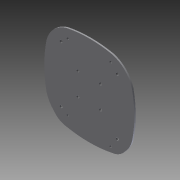
# Autodesk Inventor part: Base
Saved by Autodesk Inventor 2011 SP1 (Build 150282100, 282)
## iProperties
Created: 2011-07-18
Part Number: Base
Document SubType Name: Modeling
Designer: Nathan
Density: 1 g/cm^3
Author: Nathan
Autodesk Inventor part; units mm, degrees
ref_plane "YZ Plane" through (0, 0, 0) normal (1, 0, 0) x (0, 1, 0)
ref_plane "XZ Plane" through (0, 0, 0) normal (0, 1, 0) x (-1, 0, 0)
ref_plane "XY Plane" through (0, 0, 0) normal (0, 0, 1) x (1, 0, 0)
sketch "Sketch1" plane through (0, 0, 0) normal (0, 0, 1) x (1, 0, 0)
  line L0 (0, 3.1673) -> (0, -2.4908)
  spline S0 degree 2 poles (-48.26, -25.4) (-53.34, 0) (-48.26, 25.4) knots 0 0 0 1 1 1
  line L1 (-20.5368, 0) -> (25.7294, 0)
  line L2 (0, 0) -> (-9.8402, -9.8402)
  line L3 (0, 0) -> (13.9161, 0) construction
  line L4 (0, 0) -> (-23.2805, 23.2805)
  arc A0 (-39.9068, 39.9068) -> (-48.26, 25.4) centre (-17.1376, 17.1376) ccw
  arc A1 (-48.26, -25.4) -> (-39.9068, -39.9068) centre (-17.1376, -17.1376) ccw
  spline S1 degree 2 poles (48.26, -25.4) (53.34, 0) (48.26, 25.4) knots 0 0 0 1 1 1
  arc A2 (48.26, 25.4) -> (39.9068, 39.9068) centre (17.1376, 17.1376) ccw
  arc A3 (39.9068, -39.9068) -> (48.26, -25.4) centre (17.1376, -17.1376) ccw
  spline S2 degree 2 poles (25.476, -48.26) (-0.0768, -53.34) (-25.476, -48.26) knots 0 0 0 1 1 1
  arc A4 (-39.9068, -39.9068) -> (-25.476, -48.26) centre (-23.264, -27.7968) ccw
  arc A5 (25.476, -48.26) -> (39.9068, -39.9068) centre (23.264, -27.7968) ccw
  spline S3 degree 2 poles (-25.4, 48.26) (0, 53.34) (25.4, 48.26) knots 0 0 0 1 1 1
  arc A6 (39.9068, 39.9068) -> (25.4, 48.26) centre (17.1376, 17.1376) ccw
  arc A7 (-25.4, 48.26) -> (-39.9068, 39.9068) centre (-17.1376, 17.1376) ccw
  point P0 (-50.8, 0)
  point P1 (50.8, 0)
  point P2 (-0.076, -50.8)
  point P3 (0, 50.8)
  point P4 (-12.7, 12.7)
  point P5 (-31.75, 31.75)
  point P6 (-31.75, -31.75)
  point P7 (-12.7, -12.7)
  point P8 (12.7, 12.7)
  point P9 (31.75, 31.75)
  point P10 (31.75, -31.75)
  point P11 (12.7, -12.7)
  point P12 (24.13, -42.935)
  point P13 (24.13, 39.615)
  point P14 (-24.13, 38.345)
  point P15 (-24.13, -36.585)
  dimension "d23" = 1.5875
  dimension "d24" = 0
  dimension "d1" = 45
  dimension "d6" = 50.8
  dimension "d7" = 25.4
  dimension "d8" = 48.26
  dimension "d15" = 48.26
  dimension "d16" = 50.8
  dimension "d17" = 25.4
  dimension "d19" = 25.4
  dimension "d20" = 50.8
  dimension "d21" = 48.26
  dimension "d22" = 25.4
  dimension "d25" = 12.7
  dimension "d26" = 31.75
  dimension "d34" = 48.26
  dimension "d38" = 48.26
  dimension "d39" = 6.35
  dimension "d40" = 82.55
  dimension "d41" = 1.27
  dimension "d42" = 48.26
  dimension "d43" = 0
  dimension "d44" = 24.13
  constraints: 17 symmetric about line, 16 point on circle, 10 end point, 8 centre point, 8 point on line, 2 horizontal, 2 perpendicular, 2 vertical, 1 equal length, 15 other
  measures "d1" angle of L3 L2
  measures "d6" distance from line of point (-50.8, 0) L0
  measures "d7" vertical distance of A0.end point (-50.8, 0)
  measures "d8" distance from line of A0.end L0
  measures "d15" distance from line of L1 A4.end
  measures "d16" distance from line of L1 point (-0.076, -50.8)
  measures "d17" horizontal distance of point (-0.076, -50.8) A4.end
  measures "d19" horizontal distance of A7.start point (0, 50.8)
  measures "d20" distance from line of L1 point (0, 50.8)
  measures "d21" distance from line of L1 A6.end
  measures "d22" horizontal distance of A6.end point (0, 50.8)
  measures "d25" horizontal distance of L2.start point (-12.7, 12.7)
  measures "d26" distance from line of L1 point (-31.75, 31.75)
  measures "d34" distance from line of L1 A7.start
  measures "d38" horizontal distance of point (-24.13, -36.585) point (24.13, -42.935)
  measures "d39" vertical distance of point (24.13, -42.935) point (-24.13, -36.585)
  measures "d40" distance of point (24.13, -42.935) point (24.13, 39.615)
  measures "d41" vertical distance of point (24.13, 39.615) point (-24.13, 38.345)
  measures "d42" horizontal distance of point (24.13, 39.615) point (-24.13, 38.345)
  measures "d43" horizontal distance of point (24.13, 39.615) point (24.13, -42.935)
  measures "d44" distance from line of L0 point (-24.13, 38.345)
extrude "Extrusion1" add sketch "Sketch1" along normal blind 1.5875
hole "Hole1" at (-12.7, 12.7, 0) at (-31.75, 31.75, 0) at (-31.75, -31.75, 0) at (-12.7, -12.7, 0) at (31.75, 31.75, 0) at (12.7, 12.7, 0) at (12.7, -12.7, 0) at (31.75, -31.75, 0) direction (0, 0, 1) diameter 3.302 end through all thread size "8-32 UNC" class "2B" standard "ANSI Unified Screw Threads"
hole "Hole2" at (24.13, -42.935, 0) at (24.13, 39.615, 0) at (-24.13, 38.345, 0) at (-24.13, -36.585, 0) direction (0, 0, 1) diameter 2.6416 end through all thread size "6-32 UNC" class "2B" standard "ANSI Unified Screw Threads"
equation "\"d15\" = d8"
equation "\"d16\" = d6"
equation "\"d20\" = d6"
equation "\"d21\" = d8"
body "Solid1"
